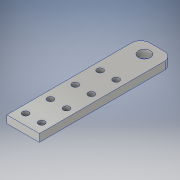
# Autodesk Inventor part: Part2_new
Saved by Autodesk Inventor 2016 (Build 200138000, 138)
## iProperties
Created: 2017-01-04
Part Number: Part2_new
Material: Aluminium 6061
Document SubType Name: Modeling
Designer: Marc
Mass: 12.1119 g
Surface Area: 33.2849 cm^2
Volume: 4.48588 cm^3
Density: 2.7 g/cm^3
Appearance: Aluminium - flach
Author: Marc
Autodesk Inventor part; units mm, degrees
ref_plane "YZ Plane" through (0, 0, 0) normal (1, 0, 0) x (0, 1, 0)
ref_plane "XZ Plane" through (0, 0, 0) normal (0, 1, 0) x (-1, 0, 0)
ref_plane "XY Plane" through (0, 0, 0) normal (0, 0, 1) x (1, 0, 0)
sketch "Skizze1" plane through (0, 0, 0) normal (0, 0, 1) x (1, 0, 0)
  line L0 (-8.5, -35) -> (8.5, -35)
  line L1 (8.5, -35) -> (8.5, 30.7574)
  line L2 (4.2574, 35) -> (-4.2574, 35)
  line L3 (-8.5, 30.7574) -> (-8.5, -35)
  line L4 (-12.1954, 0) -> (12.1954, 0) projected
  line L5 (0, -49.0422) -> (0, 49.2532) projected
  circle A0 centre (0, 28.5) radius 3.15
  circle A1 centre (-4.2, -29.5) radius 1.65
  circle A2 centre (4.2, -29.5) radius 1.65
  circle A3 centre (-4.2, -16.5) radius 1.65
  circle A4 centre (4.2, -16.5) radius 1.65
  circle A5 centre (-4.2, -3.5) radius 1.65
  circle A6 centre (4.2, -3.5) radius 1.65
  circle A7 centre (-4.2, 9.5) radius 1.65
  circle A8 centre (4.2, 9.5) radius 1.65
  line L6 (-6.3787, 34.1213) -> (-7.6213, 32.8787)
  line L7 (6.3787, 34.1213) -> (7.6213, 32.8787)
  arc A9 (8.5, 30.7574) -> (7.6213, 32.8787) centre (5.5, 30.7574) ccw
  arc A10 (6.3787, 34.1213) -> (4.2574, 35) centre (4.2574, 32) ccw
  arc A11 (-4.2574, 35) -> (-6.3787, 34.1213) centre (-4.2574, 32) ccw
  arc A12 (-7.6213, 32.8787) -> (-8.5, 30.7574) centre (-5.5, 30.7574) ccw
  point P0 (0, 0)
  point P1 (8.5, 35)
  point P2 (-8.5, 35)
  point P3 (-5.5, 35)
  point P4 (-8.5, 32)
  point P5 (5.5, 35)
  point P6 (8.5, 32)
  dimension "d0" = 17
  dimension "d1" = 70
  dimension "d2" = 6.3
  dimension "d3" = 6.5
  dimension "d4" = 3.3
  dimension "d5" = 3.3
  dimension "d6" = 3.3
  dimension "d7" = 3.3
  dimension "d8" = 3.3
  dimension "d9" = 3.3
  dimension "d10" = 3.3
  dimension "d11" = 3.3
  dimension "d12" = 4.3
  dimension "d13" = 8.4
  dimension "d14" = 5.5
  dimension "d15" = 13
  dimension "d16" = 13
  dimension "d17" = 13
  dimension "d18" = 3
  dimension "d19" = 3
  dimension "d20" = 3
  dimension "d21" = 3
  dimension "d24" = 3
  constraints: 13 centre point, 13 point on line, 12 end point, 8 point on circle, 8 tangent, 6 vertical alignment, 4 horizontal alignment, 3 equal radius, 2 parallel, 1 horizontal, 1 perpendicular, 2 other
  measures "d0" distance of point (-8.5, 35) point (8.5, 35)
  measures "d1" distance of point (8.5, 35) L0.end
  measures "d2" diameter of A0
  measures "d3" distance from line of L2 A0.centre
  measures "d4" diameter of A1
  measures "d5" diameter of A2
  measures "d6" diameter of A3
  measures "d7" diameter of A4
  measures "d8" diameter of A5
  measures "d9" diameter of A6
  measures "d10" diameter of A7
  measures "d11" diameter of A8
  measures "d12" distance from line of L3 A1.centre
  measures "d13" distance of A2.centre A1.centre
  measures "d14" distance from line of L0 A1.centre
  measures "d15" distance of A3.centre A1.centre
  measures "d16" distance of A5.centre A3.centre
  measures "d17" distance of A7.centre A5.centre
  measures "d18" distance of point (-5.5, 35) point (-8.5, 35)
  measures "d19" distance of point (-8.5, 32) point (-8.5, 35)
  measures "d20" distance of point (5.5, 35) point (8.5, 35)
  measures "d21" distance of point (8.5, 32) point (8.5, 35)
  measures "d24" radius of A9
extrude "Extrusion1" add sketch "Skizze1" along normal blind 4 contours L3 L4 L5 L0 | L5 L4 L1 L0 | L3 A12 L6 A11 L2 L5 A0 L4 | L5 A0 L2 A10 L7 A9 L1 L4
equation "\"d4\" = d5"
equation "\"d6\" = d5"
equation "\"d7\" = d5"
equation "\"d8\" = d5"
equation "\"d9\" = d5"
equation "\"d10\" = d5"
equation "\"d11\" = d5"
equation "\"d19\" = d18"
equation "\"d20\" = d18"
equation "\"d21\" = d20"
